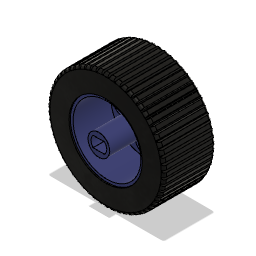
_k346tt.829baadc-af93-402c-a998-022c70149929 (Autodesk Fusion 360 design; units mm, degrees)
Autodesk Fusion 360 part; units mm, degrees
note: some values were not read from the file. Chosen so that the rebuilt part matches the saved one: which bodies a step acts on; which face or edge a step refers to. Set by a fixed rule: which sketch regions a step uses.
sketch "Sketch1" plane through (0, 0, 0) normal (0, 0, 1) x (1, 0, 0)
  circle A0 centre (0, 0) radius 17.5
  line L0 (0, -4) -> (0, -12.5)
  line L1 (12.5, 0) -> (13.5, 0) construction
  arc A1 (9.5459, 9.5459) -> (13.4629, 1) centre (0, 0) ccw
  arc A2 (-3.4457, 2.0315) -> (-4, 0) centre (0, 0) ccw
  arc A3 (-1, 3.873) -> (-2.8284, 2.8284) centre (0, 0) ccw
  arc A4 (2.0315, 3.4457) -> (0, 4) centre (0, 0) ccw
  arc A5 (3.873, 1) -> (2.8284, 2.8284) centre (0, 0) ccw
  arc A6 (3.4457, -2.0315) -> (4, 0) centre (0, 0) ccw
  arc A7 (1, -3.873) -> (2.8284, -2.8284) centre (0, 0) ccw
  arc A8 (-3.873, -1) -> (-2.8284, -2.8284) centre (0, 0) ccw
  arc A9 (-2.0315, -3.4457) -> (0, -4) centre (0, 0) ccw
  arc A10 (-12.4599, -1) -> (-8.8388, -8.8388) centre (0, 0) ccw
  arc A11 (-8.1034, -9.5176) -> (0, -12.5) centre (0, 0) ccw
  arc A12 (1, -12.4599) -> (8.8388, -8.8388) centre (0, 0) ccw
  arc A13 (9.5176, -8.1034) -> (12.5, 0) centre (0, 0) ccw
  arc A14 (12.4599, 1) -> (8.8388, 8.8388) centre (0, 0) ccw
  arc A15 (8.1034, 9.5176) -> (0, 12.5) centre (0, 0) ccw
  arc A16 (-1, 12.4599) -> (-8.8388, 8.8388) centre (0, 0) ccw
  arc A17 (-9.5176, 8.1034) -> (-12.5, 0) centre (0, 0) ccw
  circle A18 centre (0, 0) radius 4
  line L2 (-14.6351, -7.6854) -> (-14.6074, -7.6729)
  line L3 (-12.5, 0) -> (45, 0) construction
  line L4 (0, 12.5) -> (0, 4)
  arc A19 (1, -13.4629) -> (12.9431, -3.8375) centre (0, 0) ccw
  arc A20 (13.4629, 1) -> (-11.8657, -6.4386) centre (0, 0) ccw
  arc A21 (-8.8126, -10.2268) -> (0, -13.5) centre (0, 0) ccw
  line L5 (0, -1.975) -> (2.1235, -1.975)
  arc A22 (2.1235, -1.975) -> (2.1235, 1.975) centre (0, 0) ccw
  line L6 (0, 1.975) -> (2.1235, 1.975)
  line L7 (0, 1.975) -> (-2.1235, 1.975)
  arc A23 (-2.1235, 1.975) -> (-2.1235, -1.975) centre (0, 0) ccw
  line L8 (0, -1.975) -> (-2.1235, -1.975)
  circle A24 centre (0, 0) radius 1.5
  circle A25 centre (0, 0) radius 12.5
  line L9 (4, 0) -> (12.5, 0)
  line L10 (-4, 0) -> (-12.5, 0)
  line L11 (-4, 0) -> (-12.5, 0)
  line L12 (0, 4) -> (0, 12.5)
  line L13 (0, -12.5) -> (0, -4)
  circle A26 centre (0, -8.25) radius 3.5
  circle A27 centre (-8.25, 0) radius 3.5
  circle A28 centre (0, 8.25) radius 3.5
  circle A29 centre (8.25, 0) radius 3.5
  line L14 (0.904, 20.4801) -> (0.7023, 21.4885)
  line L15 (-0.7023, 21.4885) -> (-0.904, 20.4801)
  arc A30 (0.7023, 21.4885) -> (-0.7023, 21.4885) centre (0, 0) ccw
  arc A31 (-1.5858, 21.4414) -> (-2.9824, 21.2921) centre (0, 0) ccw
  line L16 (-2.9824, 21.2921) -> (-3.0758, 20.2679)
  line L17 (-1.278, 20.4601) -> (-1.5858, 21.4414)
  arc A32 (-3.8559, 21.1514) -> (-5.2287, 20.8545) centre (0, 0) ccw
  line L18 (-5.2287, 20.8545) -> (-5.2127, 19.8262)
  line L19 (-3.4456, 20.2084) -> (-3.8559, 21.1514)
  arc A33 (-6.0823, 20.6217) -> (-7.4158, 20.1806) centre (0, 0) ccw
  line L20 (-7.4158, 20.1806) -> (-7.2906, 19.1598)
  line L21 (-5.5741, 19.7276) -> (-6.0823, 20.6217)
  arc A34 (-8.2398, 19.8584) -> (-9.5189, 19.278) centre (0, 0) ccw
  line L22 (-9.5189, 19.278) -> (-9.2858, 18.2763)
  line L23 (-7.6394, 19.0234) -> (-8.2398, 19.8584)
  arc A35 (-10.3039, 18.8701) -> (-11.5141, 18.157) centre (0, 0) ccw
  line L24 (-11.5141, 18.157) -> (-11.1759, 17.1858)
  line L25 (-9.6182, 18.1036) -> (-10.3039, 18.8701)
  arc A36 (-12.2513, 17.6679) -> (-13.3788, 16.8303) centre (0, 0) ccw
  line L26 (-13.3788, 16.8303) -> (-12.9393, 15.9005)
  line L27 (-11.488, 16.9787) -> (-12.2513, 17.6679)
  arc A37 (-14.0599, 16.2656) -> (-15.092, 15.3128) centre (0, 0) ccw
  line L28 (-15.092, 15.3128) -> (-14.5561, 14.435)
  line L29 (-13.2276, 15.6614) -> (-14.0599, 16.2656)
  arc A38 (-15.7092, 14.679) -> (-16.6341, 13.6219) centre (0, 0) ccw
  line L30 (-16.6341, 13.6219) -> (-16.008, 12.806)
  line L31 (-14.8174, 14.1667) -> (-15.7092, 14.679)
  arc A39 (-17.1805, 12.926) -> (-17.9878, 11.7766) centre (0, 0) ccw
  line L32 (-17.9878, 11.7766) -> (-17.2785, 11.0319)
  line L33 (-16.2393, 12.5114) -> (-17.1805, 12.926)
  arc A40 (-18.4571, 11.0266) -> (-19.1377, 9.7979) centre (0, 0) ccw
  line L34 (-19.1377, 9.7979) -> (-18.3532, 9.1329)
  line L35 (-17.4772, 10.7144) -> (-18.4571, 11.0266)
  arc A41 (-19.5246, 9.0023) -> (-20.0707, 7.7082) centre (0, 0) ccw
  line L36 (-20.0707, 7.7082) -> (-19.22, 7.1303)
  line L37 (-18.517, 8.796) -> (-19.5246, 9.0023)
  arc A42 (-20.3708, 6.876) -> (-20.7763, 5.5312) centre (0, 0) ccw
  line L38 (-20.7763, 5.5312) -> (-19.869, 5.0469)
  line L39 (-19.3471, 6.7779) -> (-20.3708, 6.876)
  arc A43 (-20.9863, 4.6717) -> (-21.2466, 3.2914) centre (0, 0) ccw
  line L40 (-21.2466, 3.2914) -> (-20.2929, 2.9064)
  line L41 (-19.9579, 4.6831) -> (-20.9863, 4.6717)
  arc A44 (-21.364, 2.4145) -> (-21.4761, 1.0144) centre (0, 0) ccw
  line L42 (-21.4761, 1.0144) -> (-20.4869, 0.7329)
  line L43 (-20.3426, 2.5351) -> (-21.364, 2.4145)
  arc A45 (-21.4996, 0.13) -> (-21.4622, -1.2741) centre (0, 0) ccw
  line L44 (-21.4622, -1.2741) -> (-20.4487, -1.4489)
  line L45 (-20.4969, 0.3585) -> (-21.4996, 0.13)
  arc A46 (-21.3916, -2.156) -> (-21.2052, -3.5482) centre (0, 0) ccw
  line L46 (-21.2052, -3.5482) -> (-20.1789, -3.6142)
  line L47 (-20.4189, -1.8222) -> (-21.3916, -2.156)
  arc A47 (-21.0413, -4.4176) -> (-20.7079, -5.782) centre (0, 0) ccw
  line L48 (-20.7079, -5.782) -> (-19.6804, -5.7386)
  line L49 (-20.1095, -3.9823) -> (-21.0413, -4.4176)
  arc A48 (-20.4525, -6.6291) -> (-19.976, -7.9504) centre (0, 0) ccw
  line L50 (-19.976, -7.9504) -> (-18.9589, -7.798)
  line L51 (-19.5723, -6.0972) -> (-20.4525, -6.6291)
  arc A49 (-19.632, -8.7655) -> (-19.0178, -10.0287) centre (0, 0) ccw
  line L52 (-19.0178, -10.0287) -> (-18.0226, -9.769)
  line L53 (-18.8133, -8.1431) -> (-19.632, -8.7655)
  arc A50 (-18.5891, -10.8026) -> (-17.8441, -11.9933) centre (0, 0) ccw
  line L54 (-17.8441, -11.9933) -> (-16.8822, -11.6294)
  line L55 (-17.8411, -10.0967) -> (-18.5891, -10.8026)
  arc A51 (-17.3355, -12.7173) -> (-16.4681, -13.8221) centre (0, 0) ccw
  line L56 (-16.4681, -13.8221) -> (-15.5504, -13.358)
  line L57 (-16.6669, -11.9359) -> (-17.3355, -12.7173)
  arc A52 (-15.8855, -14.4879) -> (-14.9057, -15.4942) centre (0, 0) ccw
  line L58 (-14.9057, -15.4942) -> (-14.0424, -14.9352)
  line L59 (-15.3037, -13.6399) -> (-15.8855, -14.4879)
  arc A53 (-14.2556, -16.0944) -> (-13.1743, -16.9908) centre (0, 0) ccw
  line L60 (-13.1743, -16.9908) -> (-12.3754, -16.3432)
  line L61 (-13.7672, -15.1893) -> (-14.2556, -16.0944)
  arc A54 (-12.4641, -17.5185) -> (-11.2936, -18.2949) centre (0, 0) ccw
  line L62 (-11.2936, -18.2949) -> (-10.5681, -17.566)
  line L63 (-12.0747, -16.5666) -> (-12.4641, -17.5185)
  arc A55 (-10.5314, -18.7441) -> (-9.285, -19.3917) centre (0, 0) ccw
  line L64 (-9.285, -19.3917) -> (-8.641, -18.5898)
  line L65 (-10.2454, -17.7562) -> (-10.5314, -18.7441)
  arc A56 (-8.4793, -19.7573) -> (-7.1712, -20.2688) centre (0, 0) ccw
  line L66 (-7.1712, -20.2688) -> (-6.6161, -19.403)
  line L67 (-8.2999, -18.7446) -> (-8.4793, -19.7573)
  arc A57 (-6.3312, -20.5467) -> (-4.9761, -20.9162) centre (0, 0) ccw
  line L68 (-4.9761, -20.9162) -> (-4.5162, -19.9963)
  line L69 (-6.2605, -19.5207) -> (-6.3312, -20.5467)
  arc A58 (-4.1114, -21.1032) -> (-2.7247, -21.3267) centre (0, 0) ccw
  line L70 (-2.7247, -21.3267) -> (-2.3652, -20.3631)
  line L71 (-4.1501, -20.0755) -> (-4.1114, -21.1032)
  arc A59 (-1.845, -21.4207) -> (-0.4424, -21.4954) centre (0, 0) ccw
  line L72 (-0.4424, -21.4954) -> (-0.1873, -20.4991)
  line L73 (-1.9927, -20.4029) -> (-1.845, -21.4207)
  arc A60 (0.4424, -21.4954) -> (1.845, -21.4207) centre (0, 0) ccw
  line L74 (1.845, -21.4207) -> (1.9927, -20.4029)
  line L75 (0.1873, -20.4991) -> (0.4424, -21.4954)
  arc A61 (2.7247, -21.3267) -> (4.1114, -21.1032) centre (0, 0) ccw
  line L76 (4.1114, -21.1032) -> (4.1501, -20.0755)
  line L77 (2.3652, -20.3631) -> (2.7247, -21.3267)
  arc A62 (4.9761, -20.9162) -> (6.3312, -20.5467) centre (0, 0) ccw
  line L78 (6.3312, -20.5467) -> (6.2605, -19.5207)
  line L79 (4.5162, -19.9963) -> (4.9761, -20.9162)
  arc A63 (7.1712, -20.2688) -> (8.4793, -19.7573) centre (0, 0) ccw
  line L80 (8.4793, -19.7573) -> (8.2999, -18.7446)
  line L81 (6.6161, -19.403) -> (7.1712, -20.2688)
  arc A64 (9.285, -19.3917) -> (10.5314, -18.7441) centre (0, 0) ccw
  line L82 (10.5314, -18.7441) -> (10.2454, -17.7562)
  line L83 (8.641, -18.5898) -> (9.285, -19.3917)
  arc A65 (11.2936, -18.2949) -> (12.4641, -17.5185) centre (0, 0) ccw
  line L84 (12.4641, -17.5185) -> (12.0747, -16.5666)
  line L85 (10.5681, -17.566) -> (11.2936, -18.2949)
  arc A66 (13.1743, -16.9908) -> (14.2556, -16.0944) centre (0, 0) ccw
  line L86 (14.2556, -16.0944) -> (13.7672, -15.1893)
  line L87 (12.3754, -16.3432) -> (13.1743, -16.9908)
  arc A67 (14.9057, -15.4942) -> (15.8855, -14.4879) centre (0, 0) ccw
  line L88 (15.8855, -14.4879) -> (15.3037, -13.6399)
  line L89 (14.0424, -14.9352) -> (14.9057, -15.4942)
  arc A68 (16.4681, -13.8221) -> (17.3355, -12.7173) centre (0, 0) ccw
  line L90 (17.3355, -12.7173) -> (16.6669, -11.9359)
  line L91 (15.5504, -13.358) -> (16.4681, -13.8221)
  arc A69 (17.8441, -11.9933) -> (18.5891, -10.8026) centre (0, 0) ccw
  line L92 (18.5891, -10.8026) -> (17.8411, -10.0967)
  line L93 (16.8822, -11.6294) -> (17.8441, -11.9933)
  arc A70 (19.0178, -10.0287) -> (19.632, -8.7655) centre (0, 0) ccw
  line L94 (19.632, -8.7655) -> (18.8133, -8.1431)
  line L95 (18.0226, -9.769) -> (19.0178, -10.0287)
  arc A71 (19.976, -7.9504) -> (20.4525, -6.6291) centre (0, 0) ccw
  line L96 (20.4525, -6.6291) -> (19.5723, -6.0972)
  line L97 (18.9589, -7.798) -> (19.976, -7.9504)
  arc A72 (20.7079, -5.782) -> (21.0413, -4.4176) centre (0, 0) ccw
  line L98 (21.0413, -4.4176) -> (20.1095, -3.9823)
  line L99 (19.6804, -5.7386) -> (20.7079, -5.782)
  arc A73 (21.2052, -3.5482) -> (21.3916, -2.156) centre (0, 0) ccw
  line L100 (21.3916, -2.156) -> (20.4189, -1.8222)
  line L101 (20.1789, -3.6142) -> (21.2052, -3.5482)
  arc A74 (21.4622, -1.2741) -> (21.4996, 0.13) centre (0, 0) ccw
  line L102 (21.4996, 0.13) -> (20.4969, 0.3585)
  line L103 (20.4487, -1.4489) -> (21.4622, -1.2741)
  arc A75 (21.4761, 1.0144) -> (21.364, 2.4145) centre (0, 0) ccw
  line L104 (21.364, 2.4145) -> (20.3426, 2.5351)
  line L105 (20.4869, 0.7329) -> (21.4761, 1.0144)
  arc A76 (21.2466, 3.2914) -> (20.9863, 4.6717) centre (0, 0) ccw
  line L106 (20.9863, 4.6717) -> (19.9579, 4.6831)
  line L107 (20.2929, 2.9064) -> (21.2466, 3.2914)
  arc A77 (20.7763, 5.5312) -> (20.3708, 6.876) centre (0, 0) ccw
  line L108 (20.3708, 6.876) -> (19.3471, 6.7779)
  line L109 (19.869, 5.0469) -> (20.7763, 5.5312)
  arc A78 (20.0707, 7.7082) -> (19.5246, 9.0023) centre (0, 0) ccw
  line L110 (19.5246, 9.0023) -> (18.517, 8.796)
  line L111 (19.22, 7.1303) -> (20.0707, 7.7082)
  arc A79 (19.1377, 9.7979) -> (18.4571, 11.0266) centre (0, 0) ccw
  line L112 (18.4571, 11.0266) -> (17.4772, 10.7144)
  line L113 (18.3532, 9.1329) -> (19.1377, 9.7979)
  arc A80 (17.9878, 11.7766) -> (17.1805, 12.926) centre (0, 0) ccw
  line L114 (17.1805, 12.926) -> (16.2393, 12.5114)
  line L115 (17.2785, 11.0319) -> (17.9878, 11.7766)
  arc A81 (16.6341, 13.6219) -> (15.7092, 14.679) centre (0, 0) ccw
  line L116 (15.7092, 14.679) -> (14.8174, 14.1667)
  line L117 (16.008, 12.806) -> (16.6341, 13.6219)
  arc A82 (15.092, 15.3128) -> (14.0599, 16.2656) centre (0, 0) ccw
  line L118 (14.0599, 16.2656) -> (13.2276, 15.6614)
  line L119 (14.5561, 14.435) -> (15.092, 15.3128)
  arc A83 (13.3788, 16.8303) -> (12.2513, 17.6679) centre (0, 0) ccw
  line L120 (12.2513, 17.6679) -> (11.488, 16.9787)
  line L121 (12.9393, 15.9005) -> (13.3788, 16.8303)
  arc A84 (11.5141, 18.157) -> (10.3039, 18.8701) centre (0, 0) ccw
  line L122 (10.3039, 18.8701) -> (9.6182, 18.1036)
  line L123 (11.1759, 17.1858) -> (11.5141, 18.157)
  arc A85 (9.5189, 19.278) -> (8.2398, 19.8584) centre (0, 0) ccw
  line L124 (8.2398, 19.8584) -> (7.6394, 19.0234)
  line L125 (9.2858, 18.2763) -> (9.5189, 19.278)
  arc A86 (7.4158, 20.1806) -> (6.0823, 20.6217) centre (0, 0) ccw
  line L126 (6.0823, 20.6217) -> (5.5741, 19.7276)
  line L127 (7.2906, 19.1598) -> (7.4158, 20.1806)
  arc A87 (5.2287, 20.8545) -> (3.8559, 21.1514) centre (0, 0) ccw
  line L128 (3.8559, 21.1514) -> (3.4456, 20.2084)
  line L129 (5.2127, 19.8262) -> (5.2287, 20.8545)
  arc A88 (2.9824, 21.2921) -> (1.5858, 21.4414) centre (0, 0) ccw
  line L130 (1.5858, 21.4414) -> (1.278, 20.4601)
  line L131 (3.0758, 20.2679) -> (2.9824, 21.2921)
  arc A89 (5.5741, 19.7276) -> (5.2127, 19.8262) centre (0, 0) ccw
  arc A90 (7.6394, 19.0234) -> (7.2906, 19.1598) centre (0, 0) ccw
  arc A91 (9.6182, 18.1036) -> (9.2858, 18.2763) centre (0, 0) ccw
  arc A92 (11.488, 16.9787) -> (11.1759, 17.1858) centre (0, 0) ccw
  arc A93 (13.2276, 15.6614) -> (12.9393, 15.9005) centre (0, 0) ccw
  arc A94 (14.8174, 14.1667) -> (14.5561, 14.435) centre (0, 0) ccw
  arc A95 (16.2393, 12.5114) -> (16.008, 12.806) centre (0, 0) ccw
  arc A96 (17.4772, 10.7144) -> (17.2785, 11.0319) centre (0, 0) ccw
  arc A97 (18.517, 8.796) -> (18.3532, 9.1329) centre (0, 0) ccw
  arc A98 (19.3471, 6.7779) -> (19.22, 7.1303) centre (0, 0) ccw
  arc A99 (19.9579, 4.6831) -> (19.869, 5.0469) centre (0, 0) ccw
  arc A100 (20.3426, 2.5351) -> (20.2929, 2.9064) centre (0, 0) ccw
  arc A101 (20.5, 0) -> (20.4869, 0.7329) centre (0, 0) ccw
  arc A102 (20.4189, -1.8222) -> (20.4487, -1.4489) centre (0, 0) ccw
  arc A103 (20.1095, -3.9823) -> (20.1789, -3.6142) centre (0, 0) ccw
  arc A104 (19.5723, -6.0972) -> (19.6804, -5.7386) centre (0, 0) ccw
  arc A105 (18.8133, -8.1431) -> (18.9589, -7.798) centre (0, 0) ccw
  arc A106 (17.8411, -10.0967) -> (18.0226, -9.769) centre (0, 0) ccw
  arc A107 (16.6669, -11.9359) -> (16.8822, -11.6294) centre (0, 0) ccw
  arc A108 (15.3037, -13.6399) -> (15.5504, -13.358) centre (0, 0) ccw
  arc A109 (13.7672, -15.1893) -> (14.0424, -14.9352) centre (0, 0) ccw
  arc A110 (12.0747, -16.5666) -> (12.3754, -16.3432) centre (0, 0) ccw
  arc A111 (10.2454, -17.7562) -> (10.5681, -17.566) centre (0, 0) ccw
  arc A112 (8.2999, -18.7446) -> (8.641, -18.5898) centre (0, 0) ccw
  arc A113 (6.2605, -19.5207) -> (6.6161, -19.403) centre (0, 0) ccw
  arc A114 (4.1501, -20.0755) -> (4.5162, -19.9963) centre (0, 0) ccw
  arc A115 (1.9927, -20.4029) -> (2.3652, -20.3631) centre (0, 0) ccw
  arc A116 (-0.1873, -20.4991) -> (0.1873, -20.4991) centre (0, 0) ccw
  arc A117 (-2.3652, -20.3631) -> (-1.9927, -20.4029) centre (0, 0) ccw
  arc A118 (-4.5162, -19.9963) -> (-4.1501, -20.0755) centre (0, 0) ccw
  arc A119 (-6.6161, -19.403) -> (-6.2605, -19.5207) centre (0, 0) ccw
  arc A120 (-8.641, -18.5898) -> (-8.2999, -18.7446) centre (0, 0) ccw
  arc A121 (-10.5681, -17.566) -> (-10.2454, -17.7562) centre (0, 0) ccw
  arc A122 (-14.0424, -14.9352) -> (-13.7672, -15.1893) centre (0, 0) ccw
  arc A123 (-12.3754, -16.3432) -> (-12.0747, -16.5666) centre (0, 0) ccw
  arc A124 (-15.5504, -13.358) -> (-15.3037, -13.6399) centre (0, 0) ccw
  arc A125 (3.4456, 20.2084) -> (3.0758, 20.2679) centre (0, 0) ccw
  arc A126 (1.278, 20.4601) -> (0.904, 20.4801) centre (0, 0) ccw
  arc A127 (-0.904, 20.4801) -> (-1.278, 20.4601) centre (0, 0) ccw
  arc A128 (-3.0758, 20.2679) -> (-3.4456, 20.2084) centre (0, 0) ccw
  arc A129 (-5.2127, 19.8262) -> (-5.5741, 19.7276) centre (0, 0) ccw
  arc A130 (-7.2906, 19.1598) -> (-7.6394, 19.0234) centre (0, 0) ccw
  arc A131 (-9.2858, 18.2763) -> (-9.6182, 18.1036) centre (0, 0) ccw
  arc A132 (-11.1759, 17.1858) -> (-11.488, 16.9787) centre (0, 0) ccw
  arc A133 (-12.9393, 15.9005) -> (-13.2276, 15.6614) centre (0, 0) ccw
  arc A134 (-14.5561, 14.435) -> (-14.8174, 14.1667) centre (0, 0) ccw
  arc A135 (-16.8822, -11.6294) -> (-16.6669, -11.9359) centre (0, 0) ccw
  arc A136 (-18.0226, -9.769) -> (-17.8411, -10.0967) centre (0, 0) ccw
  arc A137 (-18.9589, -7.798) -> (-18.8133, -8.1431) centre (0, 0) ccw
  arc A138 (-19.6804, -5.7386) -> (-19.5723, -6.0972) centre (0, 0) ccw
  arc A139 (-20.1789, -3.6142) -> (-20.1095, -3.9823) centre (0, 0) ccw
  arc A140 (-20.4487, -1.4489) -> (-20.4189, -1.8222) centre (0, 0) ccw
  arc A141 (-20.4869, 0.7329) -> (-20.4969, 0.3585) centre (0, 0) ccw
  arc A142 (-20.2929, 2.9064) -> (-20.3426, 2.5351) centre (0, 0) ccw
  arc A143 (-19.869, 5.0469) -> (-19.9579, 4.6831) centre (0, 0) ccw
  arc A144 (-19.22, 7.1303) -> (-19.3471, 6.7779) centre (0, 0) ccw
  arc A145 (-18.3532, 9.1329) -> (-18.517, 8.796) centre (0, 0) ccw
  arc A146 (-16.008, 12.806) -> (-16.2393, 12.5114) centre (0, 0) ccw
  arc A147 (-17.2785, 11.0319) -> (-17.4772, 10.7144) centre (0, 0) ccw
  dimension "d5" = 8
  dimension "d22" = 25
  dimension "d64" = 3
  dimension "d79" = 7
  dimension "d80" = 7
  dimension "d81" = 7
  dimension "d82" = 7
  dimension "d91" = 43
  dimension "d94" = 360
  constraint coincident L0.end A10
  constraint coincident L1.start A10
  constraint coincident A15.end A10
  constraint coincident A15.start A10
  constraint coincident A14.end A10
  constraint coincident A14.start A10
  constraint coincident A13.start A10
  constraint coincident A12.end A10
  constraint coincident A6.start A8
  constraint coincident A7.start A8
  constraint coincident A9.start A8
  constraint coincident A2.start A8
  constraint coincident A3.start A8
  constraint coincident A4.start A8
  constraint coincident A5.start A8
  constraint coincident A16.start A10
  constraint coincident A16.end A10
  constraint coincident A17.start A10
  constraint coincident A11.start A10
  constraint coincident A12.start A10
  constraint concentric A2 A8
  constraint concentric A3 A8
  constraint concentric A4 A8
  constraint concentric A5 A8
  constraint concentric A6 A8
  constraint concentric A7 A8
  constraint concentric A8 A9
  constraint concentric A10 A11
  constraint concentric A11 A12
  constraint concentric A12 A14
  constraint concentric A12 A13
  constraint concentric A14 A15
  constraint concentric A15 A16
  constraint concentric A16 A17
  constraint concentric A17 A19
  constraint concentric A18 A19
  constraint coincident A1 A20.end
  constraint coincident A1 A19.end
  constraint concentric A19 A20
  constraint concentric A20 A21
  constraint horizontal L3
  constraint coincident A17.start A25
  constraint coincident A2.end L3
  constraint parallel L1 L9
  constraint parallel L4 L12
  constraint parallel L0 L13
  constraint midpoint L0 A26.centre
  constraint midpoint L11 A27.centre
  constraint midpoint L12 A28.centre
  constraint midpoint L9 A29.centre
  constraint concentric A21 A30
  constraint coincident L15.end A125
  constraint concentric A89 A125
  constraint concentric A90 A125
  constraint concentric A91 A125
  constraint concentric A92 A125
  constraint concentric A93 A125
  constraint concentric A94 A125
  constraint concentric A95 A125
  constraint concentric A96 A125
  constraint concentric A97 A125
  constraint concentric A98 A125
  constraint concentric A99 A125
  constraint concentric A100 A125
  constraint coincident L3 A101.start
  constraint concentric A101 A125
  constraint concentric A102 A125
  constraint concentric A103 A125
  constraint concentric A104 A125
  constraint concentric A105 A125
  constraint concentric A106 A125
  constraint concentric A107 A125
  constraint concentric A108 A125
  constraint concentric A109 A125
  constraint concentric A110 A125
  constraint concentric A111 A125
  constraint concentric A112 A125
  constraint concentric A113 A125
  constraint concentric A114 A125
  constraint concentric A115 A125
  constraint concentric A116 A125
  constraint concentric A117 A125
  constraint concentric A118 A125
  constraint concentric A119 A125
  constraint concentric A120 A125
  constraint concentric A121 A125
  constraint concentric A122 A125
  constraint concentric A122 A123
  constraint concentric A124 A125
  constraint concentric A125 A127
  constraint concentric A125 A126
  constraint concentric A127 A128
  constraint concentric A128 A129
  constraint concentric A129 A130
  constraint concentric A130 A131
  constraint concentric A131 A132
  constraint concentric A132 A133
  constraint concentric A133 A134
  constraint concentric A134 A146
  constraint concentric A135 A146
  constraint concentric A136 A146
  constraint concentric A137 A146
  constraint concentric A138 A146
  constraint concentric A139 A146
  constraint concentric A140 A146
  constraint concentric A141 A146
  constraint concentric A142 A146
  constraint concentric A143 A146
  constraint concentric A144 A146
  constraint concentric A145 A146
  constraint concentric A146 A147
  measures "d5" diameter of A8
  measures "d22" diameter of A10
  measures "d64" diameter of A24
  measures "d79" diameter of A26
  measures "d80" diameter of A27
  measures "d81" diameter of A28
  measures "d82" diameter of A29
  measures "d91" diameter of A30
extrude "Extrude8" add sketch "Sketch1" along normal blind 18 contours A2 A3 A4 A5 A6 A7 A8 A9 A18 | A1 A19 A20 A21 makes body 1 at (-9.7613, -9.3256, 6) makes body 2 at (3.6282, -1.684, 12)
extrude "Extrude9" add sketch "Sketch1" along normal blind 12 contours L5 A22 L6 L7 A23 L8 bodies 2
extrude "Extrude10" add sketch "Sketch1" along normal blind 4 contours L0 A6 A7 A12 A13 A18 A25 L9 L13 A26 A29 | L0 A8 A9 A10 A11 A18 A25 L10 L11 L13 A26 A27 | L0 L13 A26 | L0 L13 A26 | A2 A3 A16 A17 A18 L4 A25 L10 L11 L12 A27 A28 | A4 A5 A14 A15 A18 L4 A25 L9 L12 A28 A29 | L10 L11 A27 | L10 L11 A27 | L9 A29 | L9 A29 | L4 L12 A28 | L4 L12 A28 bodies 1 2
extrude "Extrude11" add sketch "Sketch1" along normal blind 13 contours A0 bodies 1
extrude "Extrude12" cut sketch "Sketch1" along normal blind 5 contours A0 bodies 1
chamfer "Chamfer2" distance 1.5 distance2 4 1 edges at (-16.3157, -6.3283, 5) measured on face at (17.413, -1.7424, 7.6667) on bodies 1
chamfer "Chamfer3" distance 4 distance2 1.5 1 edges at (-16.3157, -6.3283, 13) measured on face at (-16.0887, 1.2087, 13) on bodies 1
extrude "Extrude13" cut sketch "Sketch1" along normal blind 4 contours L0 L13 A26 | L0 L13 A26 | L10 L11 A27 | L10 L11 A27 | L9 A29 | L9 A29 | L4 L12 A28 | L4 L12 A28 bodies 1
extrude "Extrude15" cut sketch "Sketch1" along normal blind 21 contours A2 A3 A4 A5 A6 A7 A8 A9 A18 bodies 1 makes body 3 at (10.2772, -7.1155, 13.3333)
extrude "Extrude16" add sketch "Sketch1" along normal blind 21 contours A2 A3 A4 A5 A6 A7 A8 A9 A18 bodies 1 3
extrude "Extrude17" add sketch "Sketch1" along normal blind 19 separate body contours A0 | L14 L15 A30 A31 L16 L17 A32 L18 L19 A33 L20 L21 A34 L22 L23 A35 L24 L25 A36 L26 L27 A37 L28 L29 A38 L30 L31 A39 L32 L33 A40 L34 L35 A41 L36 L37 A42 L38 L39 A43 L40 L41 A44 L42 L43 A45 L44 L45 A46 L46 L47 A47 L48 L49 A48 L50 L51 A49 L52 L53 A50 L54 L55 A51 L56 L57 A52 L58 L59 A53 L60 L61 A54 L62 L63 A55 L64 L65 A56 L66 L67 A57 L68 L69 A58 L70 L71 A59 L72 L73 A60 L74 L75 A61 L76 L77 A62 L78 L79 A63 L80 L81 A64 L82 L83 A65 L84 L85 A66 L86 L87 A67 L88 L89 A68 L90 L91 A69 L92 L93 A70 L94 L95 A71 L96 L97 A72 L98 L99 A73 L100 L101 A74 L102 L103 A75 L104 L105 A76 L106 L107 A77 L108 L109 A78 L110 L111 A79 L112 L113 A80 L114 L115 A81 L116 L117 A82 L118 L119 A83 L120 L121 A84 L122 L123 A85 L124 L125 A86 L126 L127 A87 L128 L129 A88 L130 L131 A89 A90 A91 A92 A93 A94 A95 A96 A97 A98 A99 A100 A101 A102 A103 A104 A105 A106 A107 A108 A109 A110 A111 A112 A113 A114 A115 A116 A117 A118 A119 A120 A121 A122 A123 A124 A125 A126 A127 A128 A129 A130 A131 A132 A133 A134 A135 A136 A137 A138 A139 A140 A141 A142 A143 A144 A145 A146 A147 makes body 4
fillet "Fillet1" radius 1 35 edges at (-14.5837, 15.7976, 0) (-16.1803, 14.158, 0) (-17.5935, 12.3579, 0) (-18.8074, 10.4178, 0) (-19.8082, 8.3597, 0) (-20.5846, 6.2069, 0) (-21.1277, 3.9837, 0) (-21.4315, 1.7154, 0) (-21.4924, -0.5723, 0) (-21.3098, -2.8536, 0) (-20.8857, -5.1025, 0) (-20.2251, -7.2936, 0) (-19.3352, -9.4021, 0) (-18.2263, -11.404, 0) (-16.9109, -13.2768, 0) (-15.4038, -14.9991, 0) (-13.7222, -16.5514, 0) (-11.8852, -17.9162, 0) (-9.9135, -19.0781, 0) (-7.8295, -20.0237, 0) (-5.6567, -20.7425, 0) (-3.4199, -21.2263, 0) (-1.1443, -21.4695, 0) (1.1443, -21.4695, 0) (7.8295, -20.0237, 0) (5.6567, -20.7425, 0) (3.4199, -21.2263, 0) (9.9135, -19.0781, 0) (11.8852, -17.9162, 0) (13.7222, -16.5514, 0) (15.4038, -14.9991, 0) (16.9109, -13.2768, 0) (18.2263, -11.404, 0) (19.3352, -9.4021, 0) (20.2251, -7.2936, 0) on bodies 4
fillet "Fillet2" radius 1 20 edges at (20.8857, -5.1025, 0) (21.3098, -2.8536, 0) (21.4924, -0.5723, 0) (21.4315, 1.7154, 0) (21.1277, 3.9837, 0) (20.5846, 6.2069, 0) (19.8082, 8.3597, 0) (18.8074, 10.4178, 0) (17.5935, 12.3579, 0) (16.1803, 14.158, 0) (14.5837, 15.7976, 0) (12.8219, 17.2583, 0) (10.9148, 18.5234, 0) (8.8841, 19.5786, 0) (6.7526, 20.412, 0) (4.5447, 21.0142, 0) (2.2853, 21.3782, 0) (0, 21.5, 0) (-2.2853, 21.3782, 0) (-4.5447, 21.0142, 0) on bodies 4
fillet "Fillet3" radius 1 28 edges at (-12.8219, 17.2583, 0) (-10.9148, 18.5234, 0) (-8.8841, 19.5786, 0) (-6.7526, 20.412, 0) (-6.7526, 20.412, 19) (-8.8841, 19.5786, 19) (-10.9148, 18.5234, 19) (-12.8219, 17.2583, 19) (-4.5447, 21.0142, 19) (-2.2853, 21.3782, 19) (0, 21.5, 19) (2.2853, 21.3782, 19) (4.5447, 21.0142, 19) (6.7526, 20.412, 19) (-14.5837, 15.7976, 19) (-16.1803, 14.158, 19) (-17.5935, 12.3579, 19) (-18.8074, 10.4178, 19) (-19.8082, 8.3597, 19) (-20.5846, 6.2069, 19) (-21.1277, 3.9837, 19) (-21.4315, 1.7154, 19) (-21.4924, -0.5723, 19) (-21.3098, -2.8536, 19) (-20.8857, -5.1025, 19) (-20.2251, -7.2936, 19) (-19.3352, -9.4021, 19) (-18.2263, -11.404, 19) on bodies 4
fillet "Fillet4" radius 1 35 edges at (8.8841, 19.5786, 19) (10.9148, 18.5234, 19) (12.8219, 17.2583, 19) (14.5837, 15.7976, 19) (16.1803, 14.158, 19) (17.5935, 12.3579, 19) (18.8074, 10.4178, 19) (19.8082, 8.3597, 19) (20.5846, 6.2069, 19) (21.1277, 3.9837, 19) (21.4315, 1.7154, 19) (21.4924, -0.5723, 19) (21.3098, -2.8536, 19) (20.8857, -5.1025, 19) (20.2251, -7.2936, 19) (19.3352, -9.4021, 19) (18.2263, -11.404, 19) (-16.9109, -13.2768, 19) (-15.4038, -14.9991, 19) (-13.7222, -16.5514, 19) (-11.8852, -17.9162, 19) (-9.9135, -19.0781, 19) (-7.8295, -20.0237, 19) (-5.6567, -20.7425, 19) (-3.4199, -21.2263, 19) (-1.1443, -21.4695, 19) (1.1443, -21.4695, 19) (3.4199, -21.2263, 19) (5.6567, -20.7425, 19) (16.9109, -13.2768, 19) (7.8295, -20.0237, 19) (9.9135, -19.0781, 19) (11.8852, -17.9162, 19) (13.7222, -16.5514, 19) (15.4038, -14.9991, 19) on bodies 4
move_body "Move1" bodies 4 to x (1, 0, 0) y (0, 1, 0) z (0, 0, 1) at (0, 0, -0.5)
extrude "Extrude2" [suppressed]
extrude "Extrude3" [suppressed]
extrude "Extrude4" [suppressed]
extrude "Extrude5" [suppressed]
extrude "Extrude6" [suppressed]
extrude "Extrude7" [suppressed]
chamfer "Chamfer1" [suppressed]
named bodies: "tire"
